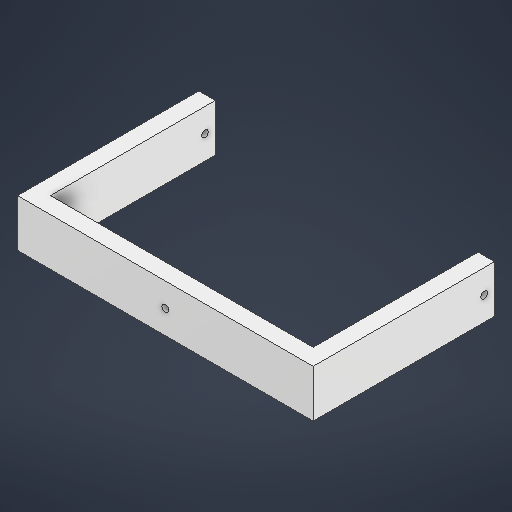
# Autodesk Inventor part: Sensor houder
Saved by Autodesk Inventor 2026.2 (Build 302298000, 298)
## iProperties
Created: 2026-05-05
Part Number: Sensor houder
Material: ABS Plastic
Document SubType Name: Modeling
Designer: Gameb
Density: 1.06 g/cm^3
Appearance: Smooth - White
Author: Gameb
Autodesk Inventor part; units mm, degrees
ref_plane "YZ Plane" through (0, 0, 0) normal (1, 0, 0) x (0, 1, 0)
ref_plane "XZ Plane" through (0, 0, 0) normal (0, 1, 0) x (-1, 0, 0)
ref_plane "XY Plane" through (0, 0, 0) normal (0, 0, 1) x (1, 0, 0)
sketch "Sketch1" plane through (0, 0, 0) normal (0, 0, 1) x (1, 0, 0)
  circle A0 centre (0, 0) radius 11.5
  circle A1 centre (0, 0) radius 1.65
  line L0 (-11.5, 0) -> (-11.5, -5)
  line L1 (-11.5, 0) -> (-11.5, 5)
  line L2 (-11.5, 5) -> (-10.3562, 5)
  line L3 (-11.5, -5) -> (-10.3562, -5)
  line L4 (11.5, 0) -> (11.5, 5)
  line L5 (11.5, 5) -> (10.3562, 5)
  line L6 (11.5, 0) -> (11.5, -5)
  line L7 (11.5, -5) -> (10.3562, -5)
  line L8 (-67.75, 0) -> (-67.75, 5)
  line L9 (-67.75, 5) -> (-11.5, 5)
  line L10 (-67.75, 0) -> (-67.75, -5)
  line L11 (-67.75, -5) -> (-11.5, -5)
  line L12 (67.75, -5) -> (67.75, 5)
  line L13 (67.75, 5) -> (11.5, 5)
  line L14 (11.5, -5) -> (67.75, -5)
  line L15 (67.75, -5) -> (71.75, -5)
  line L16 (71.75, -5) -> (71.75, 5)
  line L17 (71.75, 5) -> (67.75, 5)
  line L18 (-67.75, -5) -> (-71.75, -5)
  line L19 (-71.75, -5) -> (-71.75, 5)
  line L20 (-71.75, 5) -> (-67.75, 5)
  line L21 (0, 11.5) -> (-71.75, 11.5)
  line L22 (-71.75, 11.5) -> (-71.75, 5)
  line L23 (-71.75, -5) -> (-71.75, -11.5)
  line L24 (-71.75, -11.5) -> (0, -11.5)
  line L25 (0, -11.5) -> (71.75, -11.5)
  line L26 (71.75, -11.5) -> (71.75, -5)
  line L27 (71.75, 5) -> (71.75, 11.5)
  line L28 (0, 11.5) -> (71.75, 11.5)
  line L29 (67.75, 5) -> (67.75, 11.5)
  line L30 (67.75, 11.5) -> (63.75, 11.5)
  line L31 (63.75, 11.5) -> (63.75, -11.5)
  line L32 (-71.75, -11.5) -> (-63.75, -11.5)
  line L33 (-63.75, -11.5) -> (-63.75, 11.5)
  dimension "d0" = 23
  dimension "d1" = 3.3
  dimension "d4" = 5
  dimension "d5" = 5
  dimension "d6" = 5
  dimension "d7" = 5
  dimension "d12" = 4
  dimension "d13" = 4
  dimension "d20" = 4
  dimension "d21" = 8
  constraints: 68 end point, 16 perpendicular, 14 point on line, 6 vertical, 5 horizontal, 2 coincident, 1 centre point, 1 parallel, 10 other
  measures "d1" diameter of A1
  measures "d4" distance of L0.start L0.end
  measures "d5" distance of L0.start L1.end
  measures "d6" distance of L4.start L4.end
  measures "d7" distance of L4.start L6.end
  measures "d12" distance of L12.start L15.end
  measures "d13" distance of L10.end L18.end
  measures "d20" distance of L29.end L30.end
  measures "d21" distance of L23.end L32.end
extrude "Extrusion1" add sketch "Sketch1" along normal blind 8
extrude "Extrusion2" add sketch "Sketch1" against normal blind 80 contours L31 L28 L29 L13 | L13 L12 L14 L31 | L14 L15 L26 L25 L31 | L33 L9 L20 L22 L21 | L24 L23 L18 L11 L33 | L17 L16 L15 L12 | L29 L28 L27 L17 | L33 L11 L10 L8 L9 | L20 L8 L10 L18 L19
sketch "Sketch3" plane through (71.75, -11.5, 8) normal (1, 0, 0) x (0, 0, -1)
  line L0 (88, 23) -> (88, 0) projected
  line L1 (88, 16.4997) -> (88, 6.5022)
  line L2 (88, 6.5022) -> (2.6791, 6.5022)
  line L3 (2.6791, 6.5022) -> (2.6791, 16.4997)
  line L4 (2.6791, 16.4997) -> (88, 16.4997)
  line L5 (77.9722, 16.4997) -> (77.9722, 6.5022)
  circle A0 centre (83.0002, 11.501) radius 1.6491
  point P0 (8, 11.5)
  constraints: 10 end point, 4 point on line, 2 perpendicular, 1 centre point, 1 horizontal, 1 parallel
extrude "Extrusion4" cut sketch "Sketch3" against normal blind 200 contours A0
body "Solid1"
